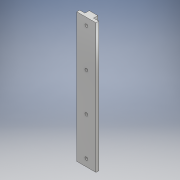
# Autodesk Inventor part: slider_b7p5x20_135_sa
Saved by Autodesk Inventor 2019 (Build 230136000, 136)
## iProperties
Created: 2018-02-23
Part Number: slider_b7p5x20_135_sa
Material: アルミニウム 6061-AHC
Document SubType Name: Modeling
Designer: shun
Density: 2.7 g/cm^3
Appearance: アルミニウム - ダーク
Author: shun
Autodesk Inventor part; units mm, degrees
ref_plane "YZ Plane" through (0, 0, 0) normal (1, 0, 0) x (0, 1, 0)
ref_plane "XZ Plane" through (0, 0, 0) normal (0, 1, 0) x (-1, 0, 0)
ref_plane "XY Plane" through (0, 0, 0) normal (0, 0, 1) x (1, 0, 0)
sketch "スケッチ1" plane through (0, 0, 0) normal (0, 0, 1) x (1, 0, 0)
  line L0 (-10, 3) -> (-4.5, 3)
  line L1 (10, 3) -> (10, 0)
  line L2 (10, 0) -> (-10, 0)
  line L3 (-10, 0) -> (-10, 3)
  line L4 (-10, 3) -> (10, 0) construction
  line L5 (10, 3) -> (-10, 0) construction
  line L6 (-4.5, 7.5) -> (4.5, 7.5)
  line L7 (4.5, 7.5) -> (4.5, 3)
  line L8 (-4.5, 3) -> (-4.5, 7.5)
  line L9 (-4.5, 7.5) -> (4.5, 3) construction
  line L10 (4.5, 7.5) -> (-4.5, 3) construction
  line L11 (4.5, 3) -> (10, 3)
  point P0 (0, 0)
  point P1 (0, 1.5)
  point P2 (0, 5.25)
  dimension "d0" = 20
  dimension "d1" = 3
  dimension "d2" = 9
  dimension "d3" = 4.5
  constraints: 24 end point, 4 midpoint, 4 parallel, 3 horizontal, 3 perpendicular, 1 point on line
  measures "d0" distance of L1.end L2.end
  measures "d1" distance of L1.start L1.end
  measures "d2" distance of L7.end L0.end
  measures "d3" distance of L6.end L7.end
extrude "押し出し1" add sketch "スケッチ1" along normal blind 135
sketch "スケッチ2" plane through (-4.5, 7.5, 0) normal (0, 1, 0) x (1, 0, 0)
  line L0 (0, 0) -> (9, 0) projected
  line L1 (9, -135) -> (0, -135) projected
  point P0 (4.5, 0)
  point P1 (4.5, -7.5)
  point P2 (4.5, -47.5)
  point P3 (4.5, -87.5)
  point P4 (4.5, -127.5)
  dimension "d6" = 7.5
  dimension "d7" = 40
  dimension "d8" = 40
  dimension "d9" = 40
  dimension "d10" = 7.5
  measures "d6" distance from line of L0 point (4.5, -7.5)
  measures "d7" distance of point (4.5, -7.5) point (4.5, -47.5)
  measures "d8" distance of point (4.5, -47.5) point (4.5, -87.5)
  measures "d9" distance of point (4.5, -127.5) point (4.5, -87.5)
  measures "d10" distance from line of L1 point (4.5, -127.5)
hole "穴1" at (0, 7.5, 7.5) at (0, 7.5, 47.5) at (0, 7.5, 87.5) at (0, 7.5, 127.5) direction (0, -1, 0) diameter 3 end through all
equation "\"d8\" = d7"
equation "\"d9\" = d7"
